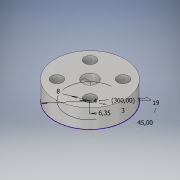
# Autodesk Inventor part: HarmonicDrive-Mounting Hub
Saved by Autodesk Inventor 2018.3 (Build 223284000, 284)
## iProperties
Created: 2018-06-25
Part Number: HarmonicDrive-Mounting Hub
Material: Generisch
Document SubType Name: Modeling
Designer: JochenAlt
Density: 1 g/cm^3
Appearance: Vorgabe
Author: JochenAlt
Autodesk Inventor part; units mm, degrees
ref_plane "YZ Plane" through (0, 0, 0) normal (1, 0, 0) x (0, 1, 0)
ref_plane "XZ Plane" through (0, 0, 0) normal (0, 1, 0) x (-1, 0, 0)
ref_plane "XY Plane" through (0, 0, 0) normal (0, 0, 1) x (1, 0, 0)
sketch "Skizze1" plane through (0, 0, 0) normal (0, 0, 1) x (1, 0, 0)
  circle A0 centre (0, 0) radius 2
  circle A1 centre (0, 0) radius 9.5
  line L0 (-13.3, 0) -> (13.3, 0) construction
  circle A2 centre (4.4901, 4.4901) radius 1.5
  circle A3 centre (-4.4901, 4.4901) radius 1.5
  circle A4 centre (-4.4901, -4.4901) radius 1.5
  circle A5 centre (4.4901, -4.4901) radius 1.5
  circle A6 centre (0, 0) radius 4
  line L1 (0, 0) -> (4.566, 4.566) construction
  dimension "d0" = 4
  dimension "d1" = 19
  dimension "d2" = 3
  dimension "d3" = 6.35
  dimension "d6" = 360
  dimension "d16" = 45
  dimension "d19" = 8
  constraints: 7 centre point, 3 coincident, 2 end point, 1 point on line, 9 other
  measures "d0" diameter of A0
  measures "d1" diameter of A1
  measures "d2" diameter of A2
  measures "d3" distance of point (0, 0) A2.centre
  measures "d16" angle of L1 L0
  measures "d19" diameter of A6
extrude "Extrusion1" add sketch "Skizze1" along normal blind 5.08 contours A1 | A6
sketch "Skizze2" plane through (0, 0, 0) normal (1, 0, 0) x (0, 1, 0)
  line L0 (0, 6.096) -> (0, -1.016) construction
  line L1 (-13.3, 0) -> (13.3, 0) construction
  circle A0 centre (0, 2.54) radius 1.5
  line L2 (9.5, 5.08) -> (-9.5, 5.08) construction
  line L3 (0, 5.08) -> (0, 0) construction
  dimension "d13" = 3
  constraints: 4 midpoint, 2 end point, 1 centre point, 1 collinear
  measures "d13" diameter of A0
extrude "Extrusion3" cut sketch "Skizze2" against normal up to surface round surface about axis through (0, 0, 0) along (0, 0, 1) radius 9.5 far side no
